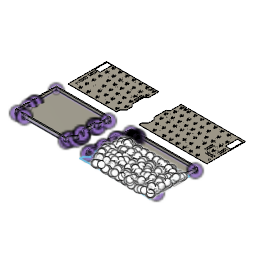
Keyboard Chassis Final v5 (Autodesk Fusion 360 design; units mm, degrees)
Autodesk Fusion 360 part; units mm, degrees
(part 1 of 12)
sketch "PCB_LEFT_MAIN" plane through (0, 0, 0) normal (0, 0, 1) x (1, 0, 0)
  line L0 (232.4105, -25.1856) -> (231.3945, -25.1856)
  line L1 (216.6624, -80.6847) -> (216.6624, -65.9527)
  line L2 (0, -1.9445) -> (0.127, -7.2798)
  line L3 (0, -79.6292) -> (0, -81.0262)
  line L4 (0, -81.0262) -> (30.2261, -80.6847)
  line L5 (231.3945, -25.1856) -> (222.2504, -16.0416)
  line L6 (0.127, -7.2798) -> (0, -32.8931)
  line L7 (222.2504, -16.0416) -> (222.2504, 39.8386)
  line L8 (233.4265, 46.9506) -> (233.4265, 92.0357)
  line L9 (226.3145, 39.8386) -> (233.4265, 46.9506)
  line L10 (222.2504, 39.8386) -> (226.3145, 39.8386)
  line L11 (232.4105, -50.2046) -> (232.4105, -25.1856)
  line L12 (233.4265, 92.0357) -> (0.635, 92.0357)
  line L13 (0.635, 92.0357) -> (0, 92.0357)
  line L14 (0, -69.7231) -> (0, -79.6292)
  line L15 (0, 92.0357) -> (0, -1.9445)
  line L16 (30.2261, -80.6847) -> (216.6624, -80.6847)
  line L17 (0, -32.8931) -> (0, -69.7231)
  line L18 (216.6624, -65.9527) -> (232.4105, -50.2046)
  line L19 (13.8092, -53.934) -> (12.9091, -53.934)
  line L20 (13.8092, -62.234) -> (12.9092, -62.234)
  line L21 (13.8092, -55.0339) -> (13.8092, -53.934)
  line L22 (13.8092, -61.1339) -> (13.8092, -62.234)
  line L23 (13.099, -61.1339) -> (13.8092, -61.1339)
  line L24 (13.8092, -55.0339) -> (13.1837, -55.0339)
  line L25 (13.1837, -55.0339) -> (13.1652, -55.0339)
  arc A0 (13.1652, -55.0339) -> (12.9092, -55.2899) centre (13.1653, -55.29) ccw
  line L26 (12.9092, -55.3429) -> (12.9092, -60.9441)
  arc A1 (12.9092, -60.9441) -> (13.099, -61.1339) centre (13.0991, -60.944) ccw
  arc A2 (13.8092, -54.1469) -> (13.8071, -54.149) centre (13.8071, -54.1469) cw
  line L27 (13.8092, -53.934) -> (12.9091, -53.934)
  line L28 (13.8092, -62.234) -> (12.9092, -62.234)
  line L29 (13.8092, -55.0339) -> (13.8092, -53.934)
  line L30 (13.8092, -61.1339) -> (13.8092, -62.234)
  line L31 (13.099, -61.1339) -> (13.8092, -61.1339)
  line L32 (13.8092, -55.0339) -> (13.1837, -55.0339)
  line L33 (13.1837, -55.0339) -> (13.1652, -55.0339)
  arc A3 (13.1652, -55.0339) -> (12.9092, -55.2899) centre (13.1653, -55.29) ccw
  line L34 (12.9092, -55.3429) -> (12.9092, -60.9441)
  arc A4 (12.9092, -60.9441) -> (13.099, -61.1339) centre (13.0991, -60.944) ccw
  arc A5 (13.8092, -54.1469) -> (13.8071, -54.149) centre (13.8071, -54.1469) cw
  arc A6 (39.6622, 82.1982) -> (43.65, 82.1982) centre (41.6561, 82.1982) ccw
  arc A7 (43.65, 82.1982) -> (39.6622, 82.1982) centre (41.6561, 82.1982) ccw
  arc A8 (47.587, 82.0712) -> (45.8852, 82.0712) centre (46.7361, 82.0712) ccw
  arc A9 (45.8852, 82.0712) -> (47.587, 82.0712) centre (46.7361, 82.0712) ccw
  arc A10 (37.427, 82.0712) -> (35.7252, 82.0712) centre (36.5761, 82.0712) ccw
  arc A11 (35.7252, 82.0712) -> (37.427, 82.0712) centre (36.5761, 82.0712) ccw
  arc A12 (69.6622, 82.1982) -> (73.65, 82.1982) centre (71.6561, 82.1982) ccw
  arc A13 (73.65, 82.1982) -> (69.6622, 82.1982) centre (71.6561, 82.1982) ccw
  arc A14 (77.587, 82.0712) -> (75.8852, 82.0712) centre (76.7361, 82.0712) ccw
  arc A15 (75.8852, 82.0712) -> (77.587, 82.0712) centre (76.7361, 82.0712) ccw
  arc A16 (65.7252, 82.0712) -> (67.427, 82.0712) centre (66.5761, 82.0712) ccw
  arc A17 (67.427, 82.0712) -> (65.7252, 82.0712) centre (66.5761, 82.0712) ccw
  arc A18 (99.6622, 82.1982) -> (103.65, 82.1982) centre (101.6561, 82.1982) ccw
  arc A19 (103.65, 82.1982) -> (99.6622, 82.1982) centre (101.6561, 82.1982) ccw
  arc A20 (107.587, 82.0712) -> (105.8852, 82.0712) centre (106.7361, 82.0712) ccw
  arc A21 (105.8852, 82.0712) -> (107.587, 82.0712) centre (106.7361, 82.0712) ccw
  arc A22 (95.7252, 82.0712) -> (97.427, 82.0712) centre (96.5761, 82.0712) ccw
  arc A23 (97.427, 82.0712) -> (95.7252, 82.0712) centre (96.5761, 82.0712) ccw
  arc A24 (133.65, 82.1982) -> (129.6622, 82.1982) centre (131.6561, 82.1982) ccw
  arc A25 (129.6622, 82.1982) -> (133.65, 82.1982) centre (131.6561, 82.1982) ccw
  arc A26 (135.8852, 82.0712) -> (137.587, 82.0712) centre (136.7361, 82.0712) ccw
  arc A27 (137.587, 82.0712) -> (135.8852, 82.0712) centre (136.7361, 82.0712) ccw
  arc A28 (125.7252, 82.0712) -> (127.427, 82.0712) centre (126.5761, 82.0712) ccw
  arc A29 (127.427, 82.0712) -> (125.7252, 82.0712) centre (126.5761, 82.0712) ccw
  arc A30 (163.65, 82.1982) -> (159.6622, 82.1982) centre (161.6561, 82.1982) ccw
  arc A31 (159.6622, 82.1982) -> (163.65, 82.1982) centre (161.6561, 82.1982) ccw
  arc A32 (167.587, 82.0712) -> (165.8852, 82.0712) centre (166.7361, 82.0712) ccw
  arc A33 (165.8852, 82.0712) -> (167.587, 82.0712) centre (166.7361, 82.0712) ccw
  arc A34 (155.7252, 82.0712) -> (157.427, 82.0712) centre (156.5761, 82.0712) ccw
  arc A35 (157.427, 82.0712) -> (155.7252, 82.0712) centre (156.5761, 82.0712) ccw
  arc A36 (193.65, 82.1982) -> (189.6622, 82.1982) centre (191.6561, 82.1982) ccw
  arc A37 (189.6622, 82.1982) -> (193.65, 82.1982) centre (191.6561, 82.1982) ccw
  arc A38 (197.587, 82.0712) -> (195.8852, 82.0712) centre (196.7361, 82.0712) ccw
  arc A39 (195.8852, 82.0712) -> (197.587, 82.0712) centre (196.7361, 82.0712) ccw
  arc A40 (187.427, 82.0712) -> (185.7252, 82.0712) centre (186.5761, 82.0712) ccw
  arc A41 (185.7252, 82.0712) -> (187.427, 82.0712) centre (186.5761, 82.0712) ccw
  arc A42 (223.65, 82.1982) -> (219.6622, 82.1982) centre (221.6561, 82.1982) ccw
  arc A43 (219.6622, 82.1982) -> (223.65, 82.1982) centre (221.6561, 82.1982) ccw
  arc A44 (227.587, 82.0712) -> (225.8852, 82.0712) centre (226.7361, 82.0712) ccw
  arc A45 (225.8852, 82.0712) -> (227.587, 82.0712) centre (226.7361, 82.0712) ccw
  arc A46 (215.7252, 82.0712) -> (217.427, 82.0712) centre (216.5761, 82.0712) ccw
  arc A47 (217.427, 82.0712) -> (215.7252, 82.0712) centre (216.5761, 82.0712) ccw
  arc A48 (39.6622, 52.1982) -> (43.65, 52.1982) centre (41.6561, 52.1982) ccw
  arc A49 (43.65, 52.1982) -> (39.6622, 52.1982) centre (41.6561, 52.1982) ccw
  arc A50 (47.587, 52.0712) -> (45.8852, 52.0712) centre (46.7361, 52.0712) ccw
  arc A51 (45.8852, 52.0712) -> (47.587, 52.0712) centre (46.7361, 52.0712) ccw
  arc A52 (37.427, 52.0712) -> (35.7252, 52.0712) centre (36.5761, 52.0712) ccw
  arc A53 (35.7252, 52.0712) -> (37.427, 52.0712) centre (36.5761, 52.0712) ccw
  arc A54 (73.65, 52.1982) -> (69.6622, 52.1982) centre (71.6561, 52.1982) ccw
  arc A55 (69.6622, 52.1982) -> (73.65, 52.1982) centre (71.6561, 52.1982) ccw
  arc A56 (75.8852, 52.0712) -> (77.587, 52.0712) centre (76.7361, 52.0712) ccw
  arc A57 (77.587, 52.0712) -> (75.8852, 52.0712) centre (76.7361, 52.0712) ccw
  arc A58 (67.427, 52.0712) -> (65.7252, 52.0712) centre (66.5761, 52.0712) ccw
  arc A59 (65.7252, 52.0712) -> (67.427, 52.0712) centre (66.5761, 52.0712) ccw
  arc A60 (103.65, 52.1982) -> (99.6622, 52.1982) centre (101.6561, 52.1982) ccw
  arc A61 (99.6622, 52.1982) -> (103.65, 52.1982) centre (101.6561, 52.1982) ccw
  arc A62 (105.8852, 52.0712) -> (107.587, 52.0712) centre (106.7361, 52.0712) ccw
  arc A63 (107.587, 52.0712) -> (105.8852, 52.0712) centre (106.7361, 52.0712) ccw
  arc A64 (97.427, 52.0712) -> (95.7252, 52.0712) centre (96.5761, 52.0712) ccw
  arc A65 (95.7252, 52.0712) -> (97.427, 52.0712) centre (96.5761, 52.0712) ccw
  arc A66 (133.65, 52.1982) -> (129.6622, 52.1982) centre (131.6561, 52.1982) ccw
  arc A67 (129.6622, 52.1982) -> (133.65, 52.1982) centre (131.6561, 52.1982) ccw
  arc A68 (137.587, 52.0712) -> (135.8852, 52.0712) centre (136.7361, 52.0712) ccw
  arc A69 (135.8852, 52.0712) -> (137.587, 52.0712) centre (136.7361, 52.0712) ccw
  arc A70 (127.427, 52.0712) -> (125.7252, 52.0712) centre (126.5761, 52.0712) ccw
  arc A71 (125.7252, 52.0712) -> (127.427, 52.0712) centre (126.5761, 52.0712) ccw
  arc A72 (159.6622, 52.1982) -> (163.65, 52.1982) centre (161.6561, 52.1982) ccw
  arc A73 (163.65, 52.1982) -> (159.6622, 52.1982) centre (161.6561, 52.1982) ccw
  arc A74 (165.8852, 52.0712) -> (167.587, 52.0712) centre (166.7361, 52.0712) ccw
  arc A75 (167.587, 52.0712) -> (165.8852, 52.0712) centre (166.7361, 52.0712) ccw
  arc A76 (155.7252, 52.0712) -> (157.427, 52.0712) centre (156.5761, 52.0712) ccw
  arc A77 (157.427, 52.0712) -> (155.7252, 52.0712) centre (156.5761, 52.0712) ccw
  arc A78 (193.65, 52.1982) -> (189.6622, 52.1982) centre (191.6561, 52.1982) ccw
  arc A79 (189.6622, 52.1982) -> (193.65, 52.1982) centre (191.6561, 52.1982) ccw
  arc A80 (197.587, 52.0712) -> (195.8852, 52.0712) centre (196.7361, 52.0712) ccw
  arc A81 (195.8852, 52.0712) -> (197.587, 52.0712) centre (196.7361, 52.0712) ccw
  arc A82 (185.7252, 52.0712) -> (187.427, 52.0712) centre (186.5761, 52.0712) ccw
  arc A83 (187.427, 52.0712) -> (185.7252, 52.0712) centre (186.5761, 52.0712) ccw
  arc A84 (219.6622, 52.1982) -> (223.65, 52.1982) centre (221.6561, 52.1982) ccw
  arc A85 (223.65, 52.1982) -> (219.6622, 52.1982) centre (221.6561, 52.1982) ccw
  arc A86 (225.8852, 52.0712) -> (227.587, 52.0712) centre (226.7361, 52.0712) ccw
  arc A87 (227.587, 52.0712) -> (225.8852, 52.0712) centre (226.7361, 52.0712) ccw
  arc A88 (217.427, 52.0712) -> (215.7252, 52.0712) centre (216.5761, 52.0712) ccw
  arc A89 (215.7252, 52.0712) -> (217.427, 52.0712) centre (216.5761, 52.0712) ccw
  arc A90 (43.65, 22.1982) -> (39.6622, 22.1982) centre (41.6561, 22.1982) ccw
  arc A91 (39.6622, 22.1982) -> (43.65, 22.1982) centre (41.6561, 22.1982) ccw
  arc A92 (45.8852, 22.0712) -> (47.587, 22.0712) centre (46.7361, 22.0712) ccw
  arc A93 (47.587, 22.0712) -> (45.8852, 22.0712) centre (46.7361, 22.0712) ccw
  arc A94 (37.427, 22.0712) -> (35.7252, 22.0712) centre (36.5761, 22.0712) ccw
  arc A95 (35.7252, 22.0712) -> (37.427, 22.0712) centre (36.5761, 22.0712) ccw
  arc A96 (75.7455, 22.2541) -> (79.7333, 22.2541) centre (77.7394, 22.2541) ccw
  arc A97 (79.7333, 22.2541) -> (75.7455, 22.2541) centre (77.7394, 22.2541) ccw
  arc A98 (83.6703, 22.1271) -> (81.9685, 22.1271) centre (82.8194, 22.1271) ccw
  arc A99 (81.9685, 22.1271) -> (83.6703, 22.1271) centre (82.8194, 22.1271) ccw
  arc A100 (73.5103, 22.1271) -> (71.8085, 22.1271) centre (72.6594, 22.1271) ccw
  arc A101 (71.8085, 22.1271) -> (73.5103, 22.1271) centre (72.6594, 22.1271) ccw
  arc A102 (105.7455, 22.2541) -> (109.7333, 22.2541) centre (107.7394, 22.2541) ccw
  arc A103 (109.7333, 22.2541) -> (105.7455, 22.2541) centre (107.7394, 22.2541) ccw
  arc A104 (111.9685, 22.1271) -> (113.6703, 22.1271) centre (112.8194, 22.1271) ccw
  arc A105 (113.6703, 22.1271) -> (111.9685, 22.1271) centre (112.8194, 22.1271) ccw
  arc A106 (101.8085, 22.1271) -> (103.5103, 22.1271) centre (102.6594, 22.1271) ccw
  arc A107 (103.5103, 22.1271) -> (101.8085, 22.1271) centre (102.6594, 22.1271) ccw
  arc A108 (135.7455, 22.2541) -> (139.7333, 22.2541) centre (137.7394, 22.2541) ccw
  arc A109 (139.7333, 22.2541) -> (135.7455, 22.2541) centre (137.7394, 22.2541) ccw
  arc A110 (143.6703, 22.1271) -> (141.9685, 22.1271) centre (142.8194, 22.1271) ccw
  arc A111 (141.9685, 22.1271) -> (143.6703, 22.1271) centre (142.8194, 22.1271) ccw
  arc A112 (133.5103, 22.1271) -> (131.8085, 22.1271) centre (132.6594, 22.1271) ccw
  arc A113 (131.8085, 22.1271) -> (133.5103, 22.1271) centre (132.6594, 22.1271) ccw
  arc A114 (165.7455, 22.2541) -> (169.7333, 22.2541) centre (167.7394, 22.2541) ccw
  arc A115 (169.7333, 22.2541) -> (165.7455, 22.2541) centre (167.7394, 22.2541) ccw
  arc A116 (173.6703, 22.1271) -> (171.9685, 22.1271) centre (172.8194, 22.1271) ccw
  arc A117 (171.9685, 22.1271) -> (173.6703, 22.1271) centre (172.8194, 22.1271) ccw
  arc A118 (163.5103, 22.1271) -> (161.8085, 22.1271) centre (162.6594, 22.1271) ccw
  arc A119 (161.8085, 22.1271) -> (163.5103, 22.1271) centre (162.6594, 22.1271) ccw
  arc A120 (199.7333, 22.2541) -> (195.7455, 22.2541) centre (197.7394, 22.2541) ccw
  arc A121 (195.7455, 22.2541) -> (199.7333, 22.2541) centre (197.7394, 22.2541) ccw
  arc A122 (203.6703, 22.1271) -> (201.9685, 22.1271) centre (202.8194, 22.1271) ccw
  arc A123 (201.9685, 22.1271) -> (203.6703, 22.1271) centre (202.8194, 22.1271) ccw
  arc A124 (193.5103, 22.1271) -> (191.8085, 22.1271) centre (192.6594, 22.1271) ccw
  arc A125 (191.8085, 22.1271) -> (193.5103, 22.1271) centre (192.6594, 22.1271) ccw
  arc A126 (118.4531, -65.1919) -> (114.4653, -65.1919) centre (116.4592, -65.1919) ccw
  arc A127 (114.4653, -65.1919) -> (118.4531, -65.1919) centre (116.4592, -65.1919) ccw
  arc A128 (122.3901, -65.3189) -> (120.6883, -65.3189) centre (121.5392, -65.3189) ccw
  arc A129 (120.6883, -65.3189) -> (122.3901, -65.3189) centre (121.5392, -65.3189) ccw
  arc A130 (112.2301, -65.3189) -> (110.5283, -65.3189) centre (111.3792, -65.3189) ccw
  arc A131 (110.5283, -65.3189) -> (112.2301, -65.3189) centre (111.3792, -65.3189) ccw
  arc A132 (39.6622, -7.8018) -> (43.65, -7.8018) centre (41.6561, -7.8018) ccw
  arc A133 (43.65, -7.8018) -> (39.6622, -7.8018) centre (41.6561, -7.8018) ccw
  arc A134 (47.587, -7.9288) -> (45.8852, -7.9288) centre (46.7361, -7.9288) ccw
  arc A135 (45.8852, -7.9288) -> (47.587, -7.9288) centre (46.7361, -7.9288) ccw
  arc A136 (37.427, -7.9288) -> (35.7252, -7.9288) centre (36.5761, -7.9288) ccw
  arc A137 (35.7252, -7.9288) -> (37.427, -7.9288) centre (36.5761, -7.9288) ccw
  arc A138 (86.6675, -7.845) -> (90.6553, -7.845) centre (88.6614, -7.845) ccw
  arc A139 (90.6553, -7.845) -> (86.6675, -7.845) centre (88.6614, -7.845) ccw
  arc A140 (94.5923, -7.972) -> (92.8905, -7.972) centre (93.7414, -7.972) ccw
  arc A141 (92.8905, -7.972) -> (94.5923, -7.972) centre (93.7414, -7.972) ccw
  arc A142 (84.4323, -7.972) -> (82.7305, -7.972) centre (83.5814, -7.972) ccw
  arc A143 (82.7305, -7.972) -> (84.4323, -7.972) centre (83.5814, -7.972) ccw
  arc A144 (116.6675, -7.845) -> (120.6553, -7.845) centre (118.6614, -7.845) ccw
  arc A145 (120.6553, -7.845) -> (116.6675, -7.845) centre (118.6614, -7.845) ccw
  arc A146 (122.8905, -7.972) -> (124.5923, -7.972) centre (123.7414, -7.972) ccw
  arc A147 (124.5923, -7.972) -> (122.8905, -7.972) centre (123.7414, -7.972) ccw
  arc A148 (112.7305, -7.972) -> (114.4323, -7.972) centre (113.5814, -7.972) ccw
  arc A149 (114.4323, -7.972) -> (112.7305, -7.972) centre (113.5814, -7.972) ccw
  arc A150 (146.6675, -7.845) -> (150.6553, -7.845) centre (148.6614, -7.845) ccw
  arc A151 (150.6553, -7.845) -> (146.6675, -7.845) centre (148.6614, -7.845) ccw
  arc A152 (154.5923, -7.972) -> (152.8905, -7.972) centre (153.7414, -7.972) ccw
  arc A153 (152.8905, -7.972) -> (154.5923, -7.972) centre (153.7414, -7.972) ccw
  arc A154 (142.7305, -7.972) -> (144.4323, -7.972) centre (143.5814, -7.972) ccw
  arc A155 (144.4323, -7.972) -> (142.7305, -7.972) centre (143.5814, -7.972) ccw
  arc A156 (176.6675, -7.845) -> (180.6553, -7.845) centre (178.6614, -7.845) ccw
  arc A157 (180.6553, -7.845) -> (176.6675, -7.845) centre (178.6614, -7.845) ccw
  arc A158 (184.5923, -7.972) -> (182.8905, -7.972) centre (183.7414, -7.972) ccw
  arc A159 (182.8905, -7.972) -> (184.5923, -7.972) centre (183.7414, -7.972) ccw
  arc A160 (174.4323, -7.972) -> (172.7305, -7.972) centre (173.5814, -7.972) ccw
  arc A161 (172.7305, -7.972) -> (174.4323, -7.972) centre (173.5814, -7.972) ccw
  arc A162 (210.6553, -7.845) -> (206.6675, -7.845) centre (208.6614, -7.845) ccw
  arc A163 (206.6675, -7.845) -> (210.6553, -7.845) centre (208.6614, -7.845) ccw
  arc A164 (212.8905, -7.972) -> (214.5923, -7.972) centre (213.7414, -7.972) ccw
  arc A165 (214.5923, -7.972) -> (212.8905, -7.972) centre (213.7414, -7.972) ccw
  arc A166 (202.7305, -7.972) -> (204.4323, -7.972) centre (203.5814, -7.972) ccw
  arc A167 (204.4323, -7.972) -> (202.7305, -7.972) centre (203.5814, -7.972) ccw
  arc A168 (158.5344, -65.1919) -> (162.5222, -65.1919) centre (160.5283, -65.1919) ccw
  arc A169 (162.5222, -65.1919) -> (158.5344, -65.1919) centre (160.5283, -65.1919) ccw
  arc A170 (166.4592, -65.3189) -> (164.7574, -65.3189) centre (165.6083, -65.3189) ccw
  arc A171 (164.7574, -65.3189) -> (166.4592, -65.3189) centre (165.6083, -65.3189) ccw
  arc A172 (156.2992, -65.3189) -> (154.5974, -65.3189) centre (155.4483, -65.3189) ccw
  arc A173 (154.5974, -65.3189) -> (156.2992, -65.3189) centre (155.4483, -65.3189) ccw
  arc A174 (39.6622, -37.8018) -> (43.65, -37.8018) centre (41.6561, -37.8018) ccw
  arc A175 (43.65, -37.8018) -> (39.6622, -37.8018) centre (41.6561, -37.8018) ccw
  arc A176 (47.587, -37.9288) -> (45.8852, -37.9288) centre (46.7361, -37.9288) ccw
  arc A177 (45.8852, -37.9288) -> (47.587, -37.9288) centre (46.7361, -37.9288) ccw
  arc A178 (37.427, -37.9288) -> (35.7252, -37.9288) centre (36.5761, -37.9288) ccw
  arc A179 (35.7252, -37.9288) -> (37.427, -37.9288) centre (36.5761, -37.9288) ccw
  arc A180 (100.1803, -37.817) -> (96.1925, -37.817) centre (98.1864, -37.817) ccw
  arc A181 (96.1925, -37.817) -> (100.1803, -37.817) centre (98.1864, -37.817) ccw
  arc A182 (102.4155, -37.944) -> (104.1173, -37.944) centre (103.2664, -37.944) ccw
  arc A183 (104.1173, -37.944) -> (102.4155, -37.944) centre (103.2664, -37.944) ccw
  arc A184 (92.2555, -37.944) -> (93.9573, -37.944) centre (93.1064, -37.944) ccw
  arc A185 (93.9573, -37.944) -> (92.2555, -37.944) centre (93.1064, -37.944) ccw
  arc A186 (130.1803, -37.817) -> (126.1925, -37.817) centre (128.1864, -37.817) ccw
  arc A187 (126.1925, -37.817) -> (130.1803, -37.817) centre (128.1864, -37.817) ccw
  arc A188 (132.4155, -37.944) -> (134.1173, -37.944) centre (133.2664, -37.944) ccw
  arc A189 (134.1173, -37.944) -> (132.4155, -37.944) centre (133.2664, -37.944) ccw
  arc A190 (122.2555, -37.944) -> (123.9573, -37.944) centre (123.1064, -37.944) ccw
  arc A191 (123.9573, -37.944) -> (122.2555, -37.944) centre (123.1064, -37.944) ccw
  arc A192 (156.1925, -37.817) -> (160.1803, -37.817) centre (158.1864, -37.817) ccw
  arc A193 (160.1803, -37.817) -> (156.1925, -37.817) centre (158.1864, -37.817) ccw
  arc A194 (162.4155, -37.944) -> (164.1173, -37.944) centre (163.2664, -37.944) ccw
  arc A195 (164.1173, -37.944) -> (162.4155, -37.944) centre (163.2664, -37.944) ccw
  arc A196 (153.9573, -37.944) -> (152.2555, -37.944) centre (153.1064, -37.944) ccw
  arc A197 (152.2555, -37.944) -> (153.9573, -37.944) centre (153.1064, -37.944) ccw
  arc A198 (190.1803, -37.817) -> (186.1925, -37.817) centre (188.1864, -37.817) ccw
  arc A199 (186.1925, -37.817) -> (190.1803, -37.817) centre (188.1864, -37.817) ccw
  arc A200 (192.4155, -37.944) -> (194.1173, -37.944) centre (193.2664, -37.944) ccw
  arc A201 (194.1173, -37.944) -> (192.4155, -37.944) centre (193.2664, -37.944) ccw
  arc A202 (183.9573, -37.944) -> (182.2555, -37.944) centre (183.1064, -37.944) ccw
  arc A203 (182.2555, -37.944) -> (183.9573, -37.944) centre (183.1064, -37.944) ccw
  arc A204 (220.1803, -37.817) -> (216.1925, -37.817) centre (218.1864, -37.817) ccw
  arc A205 (216.1925, -37.817) -> (220.1803, -37.817) centre (218.1864, -37.817) ccw
  arc A206 (222.4155, -37.944) -> (224.1173, -37.944) centre (223.2664, -37.944) ccw
  arc A207 (224.1173, -37.944) -> (222.4155, -37.944) centre (223.2664, -37.944) ccw
  arc A208 (213.9573, -37.944) -> (212.2555, -37.944) centre (213.1064, -37.944) ccw
  arc A209 (212.2555, -37.944) -> (213.9573, -37.944) centre (213.1064, -37.944) ccw
  arc A210 (206.9723, -65.1919) -> (202.9845, -65.1919) centre (204.9784, -65.1919) ccw
  arc A211 (202.9845, -65.1919) -> (206.9723, -65.1919) centre (204.9784, -65.1919) ccw
  arc A212 (209.2075, -65.3189) -> (210.9093, -65.3189) centre (210.0584, -65.3189) ccw
  arc A213 (210.9093, -65.3189) -> (209.2075, -65.3189) centre (210.0584, -65.3189) ccw
  arc A214 (200.7493, -65.3189) -> (199.0475, -65.3189) centre (199.8984, -65.3189) ccw
  arc A215 (199.0475, -65.3189) -> (200.7493, -65.3189) centre (199.8984, -65.3189) ccw
  arc A216 (39.6622, -65.1919) -> (43.65, -65.1919) centre (41.6561, -65.1919) ccw
  arc A217 (43.65, -65.1919) -> (39.6622, -65.1919) centre (41.6561, -65.1919) ccw
  arc A218 (45.8852, -65.3189) -> (47.587, -65.3189) centre (46.7361, -65.3189) ccw
  arc A219 (47.587, -65.3189) -> (45.8852, -65.3189) centre (46.7361, -65.3189) ccw
  arc A220 (35.7252, -65.3189) -> (37.427, -65.3189) centre (36.5761, -65.3189) ccw
  arc A221 (37.427, -65.3189) -> (35.7252, -65.3189) centre (36.5761, -65.3189) ccw
  arc A222 (73.8252, -65.1919) -> (77.8131, -65.1919) centre (75.8192, -65.1919) ccw
  arc A223 (77.8131, -65.1919) -> (73.8252, -65.1919) centre (75.8192, -65.1919) ccw
  arc A224 (80.0483, -65.3189) -> (81.7501, -65.3189) centre (80.8992, -65.3189) ccw
  arc A225 (81.7501, -65.3189) -> (80.0483, -65.3189) centre (80.8992, -65.3189) ccw
  arc A226 (71.59, -65.3189) -> (69.8882, -65.3189) centre (70.7391, -65.3189) ccw
  arc A227 (69.8882, -65.3189) -> (71.59, -65.3189) centre (70.7391, -65.3189) ccw
  arc A228 (207.6588, 87.4842) -> (206.1588, 87.4842) centre (206.9088, 87.4842) ccw
  arc A229 (206.1588, 87.4842) -> (207.6588, 87.4842) centre (206.9088, 87.4842) ccw
  arc A230 (207.7096, 80.4662) -> (206.2096, 80.4662) centre (206.9596, 80.4662) ccw
  arc A231 (206.2096, 80.4662) -> (207.7096, 80.4662) centre (206.9596, 80.4662) ccw
  line L35 (43.6781, 75.6042) -> (39.8781, 75.6042)
  line L36 (39.8781, 79.4042) -> (43.6781, 79.4042)
  line L37 (43.6781, 79.4042) -> (43.6781, 75.6042)
  line L38 (39.8781, 75.6042) -> (39.8781, 79.4042)
  line L39 (69.8781, 79.4042) -> (73.6781, 79.4042)
  line L40 (69.8781, 75.6042) -> (69.8781, 79.4042)
  line L41 (73.6781, 75.6042) -> (69.8781, 75.6042)
  line L42 (73.6781, 79.4042) -> (73.6781, 75.6042)
  line L43 (99.8781, 79.4042) -> (103.6781, 79.4042)
  line L44 (103.6781, 75.6042) -> (99.8781, 75.6042)
  line L45 (103.6781, 79.4042) -> (103.6781, 75.6042)
  line L46 (99.8781, 75.6042) -> (99.8781, 79.4042)
  line L47 (129.8781, 79.4042) -> (133.6781, 79.4042)
  line L48 (129.8781, 75.6042) -> (129.8781, 79.4042)
  line L49 (133.6781, 79.4042) -> (133.6781, 75.6042)
  line L50 (133.6781, 75.6042) -> (129.8781, 75.6042)
  line L51 (163.6781, 75.6042) -> (159.8781, 75.6042)
  line L52 (159.8781, 79.4042) -> (163.6781, 79.4042)
  line L53 (159.8781, 75.6042) -> (159.8781, 79.4042)
  line L54 (163.6781, 79.4042) -> (163.6781, 75.6042)
  line L55 (189.8781, 75.6042) -> (189.8781, 79.4042)
  line L56 (193.6781, 75.6042) -> (189.8781, 75.6042)
  line L57 (193.6781, 79.4042) -> (193.6781, 75.6042)
  line L58 (189.8781, 79.4042) -> (193.6781, 79.4042)
  line L59 (219.8781, 75.6042) -> (219.8781, 79.4042)
  line L60 (223.6781, 75.6042) -> (219.8781, 75.6042)
  line L61 (223.6781, 79.4042) -> (223.6781, 75.6042)
  line L62 (219.8781, 79.4042) -> (223.6781, 79.4042)
  line L63 (43.6781, 45.6042) -> (39.8781, 45.6042)
  line L64 (43.6781, 49.4042) -> (43.6781, 45.6042)
  line L65 (39.8781, 49.4042) -> (43.6781, 49.4042)
  line L66 (39.8781, 45.6042) -> (39.8781, 49.4042)
  line L67 (73.6781, 49.4042) -> (73.6781, 45.6042)
  line L68 (69.8781, 45.6042) -> (69.8781, 49.4042)
  line L69 (69.8781, 49.4042) -> (73.6781, 49.4042)
  line L70 (73.6781, 45.6042) -> (69.8781, 45.6042)
  line L71 (103.6781, 49.4042) -> (103.6781, 45.6042)
  line L72 (99.8781, 49.4042) -> (103.6781, 49.4042)
  line L73 (99.8781, 45.6042) -> (99.8781, 49.4042)
  line L74 (103.6781, 45.6042) -> (99.8781, 45.6042)
  line L75 (129.8781, 45.6042) -> (129.8781, 49.4042)
  line L76 (133.6781, 49.4042) -> (133.6781, 45.6042)
  line L77 (133.6781, 45.6042) -> (129.8781, 45.6042)
  line L78 (129.8781, 49.4042) -> (133.6781, 49.4042)
  line L79 (159.8781, 49.4042) -> (163.6781, 49.4042)
  line L80 (163.6781, 45.6042) -> (159.8781, 45.6042)
  line L81 (159.8781, 45.6042) -> (159.8781, 49.4042)
  line L82 (163.6781, 49.4042) -> (163.6781, 45.6042)
  line L83 (189.8781, 45.6042) -> (189.8781, 49.4042)
  line L84 (193.6781, 45.6042) -> (189.8781, 45.6042)
  line L85 (189.8781, 49.4042) -> (193.6781, 49.4042)
  line L86 (193.6781, 49.4042) -> (193.6781, 45.6042)
  line L87 (223.6781, 45.6042) -> (219.8781, 45.6042)
  line L88 (219.8781, 45.6042) -> (219.8781, 49.4042)
  line L89 (223.6781, 49.4042) -> (223.6781, 45.6042)
  line L90 (219.8781, 49.4042) -> (223.6781, 49.4042)
  line L91 (43.6781, 19.4042) -> (43.6781, 15.6042)
  line L92 (39.8781, 15.6042) -> (39.8781, 19.4042)
  line L93 (43.6781, 15.6042) -> (39.8781, 15.6042)
  line L94 (39.8781, 19.4042) -> (43.6781, 19.4042)
  line L95 (75.9614, 19.4601) -> (79.7614, 19.4601)
  line L96 (79.7614, 19.4601) -> (79.7614, 15.6601)
  line L97 (79.7614, 15.6601) -> (75.9614, 15.6601)
  line L98 (75.9614, 15.6601) -> (75.9614, 19.4601)
  line L99 (109.7614, 15.6601) -> (105.9614, 15.6601)
  line L100 (105.9614, 15.6601) -> (105.9614, 19.4601)
  line L101 (109.7614, 19.4601) -> (109.7614, 15.6601)
  line L102 (105.9614, 19.4601) -> (109.7614, 19.4601)
  line L103 (135.9614, 15.6601) -> (135.9614, 19.4601)
  line L104 (139.7614, 19.4601) -> (139.7614, 15.6601)
  line L105 (139.7614, 15.6601) -> (135.9614, 15.6601)
  line L106 (135.9614, 19.4601) -> (139.7614, 19.4601)
  line L107 (165.9614, 15.6601) -> (165.9614, 19.4601)
  line L108 (169.7614, 15.6601) -> (165.9614, 15.6601)
  line L109 (169.7614, 19.4601) -> (169.7614, 15.6601)
  line L110 (165.9614, 19.4601) -> (169.7614, 19.4601)
  line L111 (199.7614, 15.6601) -> (195.9614, 15.6601)
  line L112 (195.9614, 19.4601) -> (199.7614, 19.4601)
  line L113 (195.9614, 15.6601) -> (195.9614, 19.4601)
  line L114 (199.7614, 19.4601) -> (199.7614, 15.6601)
  line L115 (114.6812, -67.9859) -> (118.4812, -67.9859)
  line L116 (114.6812, -71.7859) -> (114.6812, -67.9859)
  line L117 (118.4812, -71.7859) -> (114.6812, -71.7859)
  line L118 (118.4812, -67.9859) -> (118.4812, -71.7859)
  line L119 (39.8781, -14.3958) -> (39.8781, -10.5958)
  line L120 (43.6781, -14.3958) -> (39.8781, -14.3958)
  line L121 (43.6781, -10.5958) -> (43.6781, -14.3958)
  line L122 (39.8781, -10.5958) -> (43.6781, -10.5958)
  line L123 (86.8834, -14.439) -> (86.8834, -10.639)
  line L124 (90.6834, -14.439) -> (86.8834, -14.439)
  line L125 (86.8834, -10.639) -> (90.6834, -10.639)
  line L126 (90.6834, -10.639) -> (90.6834, -14.439)
  line L127 (120.6834, -10.639) -> (120.6834, -14.439)
  line L128 (116.8834, -14.439) -> (116.8834, -10.639)
  line L129 (120.6834, -14.439) -> (116.8834, -14.439)
  line L130 (116.8834, -10.639) -> (120.6834, -10.639)
  line L131 (146.8834, -14.439) -> (146.8834, -10.639)
  line L132 (150.6834, -10.639) -> (150.6834, -14.439)
  line L133 (146.8834, -10.639) -> (150.6834, -10.639)
  line L134 (150.6834, -14.439) -> (146.8834, -14.439)
  line L135 (180.6834, -14.439) -> (176.8834, -14.439)
  line L136 (180.6834, -10.639) -> (180.6834, -14.439)
  line L137 (176.8834, -10.639) -> (180.6834, -10.639)
  line L138 (176.8834, -14.439) -> (176.8834, -10.639)
  line L139 (206.8834, -14.439) -> (206.8834, -10.639)
  line L140 (206.8834, -10.639) -> (210.6834, -10.639)
  line L141 (210.6834, -10.639) -> (210.6834, -14.439)
  line L142 (210.6834, -14.439) -> (206.8834, -14.439)
  line L143 (158.7503, -67.9859) -> (162.5503, -67.9859)
  line L144 (158.7503, -71.7859) -> (158.7503, -67.9859)
  line L145 (162.5503, -71.7859) -> (158.7503, -71.7859)
  line L146 (162.5503, -67.9859) -> (162.5503, -71.7859)
  line L147 (39.8781, -44.3958) -> (39.8781, -40.5958)
  line L148 (43.6781, -40.5958) -> (43.6781, -44.3958)
  line L149 (43.6781, -44.3958) -> (39.8781, -44.3958)
  line L150 (39.8781, -40.5958) -> (43.6781, -40.5958)
  line L151 (96.4084, -44.411) -> (96.4084, -40.611)
  line L152 (100.2084, -40.611) -> (100.2084, -44.411)
  line L153 (100.2084, -44.411) -> (96.4084, -44.411)
  line L154 (96.4084, -40.611) -> (100.2084, -40.611)
  line L155 (126.4084, -44.411) -> (126.4084, -40.611)
  line L156 (130.2084, -44.411) -> (126.4084, -44.411)
  line L157 (126.4084, -40.611) -> (130.2084, -40.611)
  line L158 (130.2084, -40.611) -> (130.2084, -44.411)
  line L159 (156.4084, -40.611) -> (160.2084, -40.611)
  line L160 (160.2084, -44.411) -> (156.4084, -44.411)
  line L161 (156.4084, -44.411) -> (156.4084, -40.611)
  line L162 (160.2084, -40.611) -> (160.2084, -44.411)
  line L163 (190.2084, -44.411) -> (186.4084, -44.411)
  line L164 (186.4084, -44.411) -> (186.4084, -40.611)
  line L165 (186.4084, -40.611) -> (190.2084, -40.611)
  line L166 (190.2084, -40.611) -> (190.2084, -44.411)
  line L167 (216.4084, -44.411) -> (216.4084, -40.611)
  line L168 (220.2084, -44.411) -> (216.4084, -44.411)
  line L169 (220.2084, -40.611) -> (220.2084, -44.411)
  line L170 (216.4084, -40.611) -> (220.2084, -40.611)
  line L171 (207.0004, -67.9859) -> (207.0004, -71.7859)
  line L172 (203.2004, -67.9859) -> (207.0004, -67.9859)
  line L173 (207.0004, -71.7859) -> (203.2004, -71.7859)
  line L174 (203.2004, -71.7859) -> (203.2004, -67.9859)
  line L175 (39.8781, -67.9859) -> (43.6781, -67.9859)
  line L176 (43.6781, -67.9859) -> (43.6781, -71.7859)
  line L177 (43.6781, -71.7859) -> (39.8781, -71.7859)
  line L178 (39.8781, -71.7859) -> (39.8781, -67.9859)
  line L179 (77.8411, -67.9859) -> (77.8411, -71.7859)
  line L180 (74.0411, -71.7859) -> (74.0411, -67.9859)
  line L181 (77.8411, -71.7859) -> (74.0411, -71.7859)
  line L182 (74.0411, -67.9859) -> (77.8411, -67.9859)
  line L183 (7.15, 86.5354) -> (5.55, 86.5354)
  line L184 (7.15, 88.1354) -> (7.15, 86.5354)
  line L185 (5.55, 88.1354) -> (7.15, 88.1354)
  line L186 (5.55, 86.5354) -> (5.55, 88.1354)
  line L187 (5.55, 88.1354) -> (7.15, 88.1354)
  line L188 (5.55, 86.5354) -> (5.55, 88.1354)
  line L189 (7.15, 88.1354) -> (7.15, 86.5354)
  line L190 (7.15, 86.5354) -> (5.55, 86.5354)
  line L191 (5.55, 86.5354) -> (5.55, 88.1354)
  line L192 (5.55, 88.1354) -> (7.15, 88.1354)
  line L193 (7.15, 88.1354) -> (7.15, 86.5354)
  line L194 (7.15, 86.5354) -> (5.55, 86.5354)
  arc A232 (5.55, 84.7954) -> (7.15, 84.7954) centre (6.35, 84.7954) ccw
  arc A233 (7.15, 84.7954) -> (5.55, 84.7954) centre (6.35, 84.7954) ccw
  arc A234 (5.55, 84.7954) -> (7.15, 84.7954) centre (6.35, 84.7954) ccw
  arc A235 (7.15, 84.7954) -> (5.55, 84.7954) centre (6.35, 84.7954) ccw
  arc A236 (5.55, 84.7954) -> (7.15, 84.7954) centre (6.35, 84.7954) ccw
  arc A237 (7.15, 84.7954) -> (5.55, 84.7954) centre (6.35, 84.7954) ccw
  arc A238 (5.55, 82.2554) -> (7.15, 82.2554) centre (6.35, 82.2554) ccw
  arc A239 (7.15, 82.2554) -> (5.55, 82.2554) centre (6.35, 82.2554) ccw
  arc A240 (5.55, 82.2554) -> (7.15, 82.2554) centre (6.35, 82.2554) ccw
  arc A241 (7.15, 82.2554) -> (5.55, 82.2554) centre (6.35, 82.2554) ccw
  arc A242 (5.55, 82.2554) -> (7.15, 82.2554) centre (6.35, 82.2554) ccw
  arc A243 (7.15, 82.2554) -> (5.55, 82.2554) centre (6.35, 82.2554) ccw
  arc A244 (5.55, 79.7154) -> (7.15, 79.7154) centre (6.35, 79.7154) ccw
  arc A245 (7.15, 79.7154) -> (5.55, 79.7154) centre (6.35, 79.7154) ccw
  arc A246 (5.55, 79.7154) -> (7.15, 79.7154) centre (6.35, 79.7154) ccw
  arc A247 (7.15, 79.7154) -> (5.55, 79.7154) centre (6.35, 79.7154) ccw
  arc A248 (7.15, 79.7154) -> (5.55, 79.7154) centre (6.35, 79.7154) ccw
  arc A249 (5.55, 79.7154) -> (7.15, 79.7154) centre (6.35, 79.7154) ccw
  arc A250 (7.15, 77.1754) -> (5.55, 77.1754) centre (6.35, 77.1754) ccw
  arc A251 (5.55, 77.1754) -> (7.15, 77.1754) centre (6.35, 77.1754) ccw
  arc A252 (7.15, 77.1754) -> (5.55, 77.1754) centre (6.35, 77.1754) ccw
  arc A253 (5.55, 77.1754) -> (7.15, 77.1754) centre (6.35, 77.1754) ccw
  arc A254 (5.55, 77.1754) -> (7.15, 77.1754) centre (6.35, 77.1754) ccw
  arc A255 (7.15, 77.1754) -> (5.55, 77.1754) centre (6.35, 77.1754) ccw
  arc A256 (7.15, 74.6354) -> (5.55, 74.6354) centre (6.35, 74.6354) ccw
  arc A257 (5.55, 74.6354) -> (7.15, 74.6354) centre (6.35, 74.6354) ccw
  arc A258 (7.15, 74.6354) -> (5.55, 74.6354) centre (6.35, 74.6354) ccw
  arc A259 (5.55, 74.6354) -> (7.15, 74.6354) centre (6.35, 74.6354) ccw
  arc A260 (5.55, 74.6354) -> (7.15, 74.6354) centre (6.35, 74.6354) ccw
  arc A261 (7.15, 74.6354) -> (5.55, 74.6354) centre (6.35, 74.6354) ccw
  arc A262 (5.55, 72.0954) -> (7.15, 72.0954) centre (6.35, 72.0954) ccw
  arc A263 (7.15, 72.0954) -> (5.55, 72.0954) centre (6.35, 72.0954) ccw
  arc A264 (5.55, 72.0954) -> (7.15, 72.0954) centre (6.35, 72.0954) ccw
  arc A265 (7.15, 72.0954) -> (5.55, 72.0954) centre (6.35, 72.0954) ccw
  arc A266 (7.15, 72.0954) -> (5.55, 72.0954) centre (6.35, 72.0954) ccw
  arc A267 (5.55, 72.0954) -> (7.15, 72.0954) centre (6.35, 72.0954) ccw
  arc A268 (5.55, 69.5553) -> (7.15, 69.5553) centre (6.35, 69.5553) ccw
  arc A269 (7.15, 69.5553) -> (5.55, 69.5553) centre (6.35, 69.5553) ccw
  arc A270 (5.55, 69.5553) -> (7.15, 69.5553) centre (6.35, 69.5553) ccw
  arc A271 (7.15, 69.5553) -> (5.55, 69.5553) centre (6.35, 69.5553) ccw
  arc A272 (7.15, 69.5553) -> (5.55, 69.5553) centre (6.35, 69.5553) ccw
  arc A273 (5.55, 69.5553) -> (7.15, 69.5553) centre (6.35, 69.5553) ccw
  arc A274 (7.15, 67.0153) -> (5.55, 67.0153) centre (6.35, 67.0153) ccw
  arc A275 (5.55, 67.0153) -> (7.15, 67.0153) centre (6.35, 67.0153) ccw
  arc A276 (7.15, 67.0153) -> (5.55, 67.0153) centre (6.35, 67.0153) ccw
  arc A277 (5.55, 67.0153) -> (7.15, 67.0153) centre (6.35, 67.0153) ccw
  arc A278 (7.15, 67.0153) -> (5.55, 67.0153) centre (6.35, 67.0153) ccw
  arc A279 (5.55, 67.0153) -> (7.15, 67.0153) centre (6.35, 67.0153) ccw
  arc A280 (5.55, 64.4753) -> (7.15, 64.4753) centre (6.35, 64.4753) ccw
  arc A281 (7.15, 64.4753) -> (5.55, 64.4753) centre (6.35, 64.4753) ccw
  arc A282 (5.55, 64.4753) -> (7.15, 64.4753) centre (6.35, 64.4753) ccw
  arc A283 (7.15, 64.4753) -> (5.55, 64.4753) centre (6.35, 64.4753) ccw
  arc A284 (7.15, 64.4753) -> (5.55, 64.4753) centre (6.35, 64.4753) ccw
  arc A285 (5.55, 64.4753) -> (7.15, 64.4753) centre (6.35, 64.4753) ccw
  arc A286 (5.55, 61.9353) -> (7.15, 61.9353) centre (6.35, 61.9353) ccw
  arc A287 (7.15, 61.9353) -> (5.55, 61.9353) centre (6.35, 61.9353) ccw
  arc A288 (5.55, 61.9353) -> (7.15, 61.9353) centre (6.35, 61.9353) ccw
  arc A289 (7.15, 61.9353) -> (5.55, 61.9353) centre (6.35, 61.9353) ccw
  arc A290 (7.15, 61.9353) -> (5.55, 61.9353) centre (6.35, 61.9353) ccw
  arc A291 (5.55, 61.9353) -> (7.15, 61.9353) centre (6.35, 61.9353) ccw
  arc A292 (5.55, 59.3953) -> (7.15, 59.3953) centre (6.35, 59.3953) ccw
  arc A293 (7.15, 59.3953) -> (5.55, 59.3953) centre (6.35, 59.3953) ccw
  arc A294 (5.55, 59.3953) -> (7.15, 59.3953) centre (6.35, 59.3953) ccw
  arc A295 (7.15, 59.3953) -> (5.55, 59.3953) centre (6.35, 59.3953) ccw
  arc A296 (7.15, 59.3953) -> (5.55, 59.3953) centre (6.35, 59.3953) ccw
  arc A297 (5.55, 59.3953) -> (7.15, 59.3953) centre (6.35, 59.3953) ccw
  arc A298 (5.55, 56.8553) -> (7.15, 56.8553) centre (6.35, 56.8553) ccw
  arc A299 (7.15, 56.8553) -> (5.55, 56.8553) centre (6.35, 56.8553) ccw
  arc A300 (7.15, 56.8553) -> (5.55, 56.8553) centre (6.35, 56.8553) ccw
  arc A301 (5.55, 56.8553) -> (7.15, 56.8553) centre (6.35, 56.8553) ccw
  arc A302 (5.55, 56.8553) -> (7.15, 56.8553) centre (6.35, 56.8553) ccw
  arc A303 (7.15, 56.8553) -> (5.55, 56.8553) centre (6.35, 56.8553) ccw
  arc A304 (5.55, 54.3153) -> (7.15, 54.3153) centre (6.35, 54.3153) ccw
  arc A305 (7.15, 54.3153) -> (5.55, 54.3153) centre (6.35, 54.3153) ccw
  arc A306 (7.15, 54.3153) -> (5.55, 54.3153) centre (6.35, 54.3153) ccw
  arc A307 (5.55, 54.3153) -> (7.15, 54.3153) centre (6.35, 54.3153) ccw
  arc A308 (5.55, 54.3153) -> (7.15, 54.3153) centre (6.35, 54.3153) ccw
  arc A309 (7.15, 54.3153) -> (5.55, 54.3153) centre (6.35, 54.3153) ccw
  arc A310 (5.55, 51.7753) -> (7.15, 51.7753) centre (6.35, 51.7753) ccw
  arc A311 (7.15, 51.7753) -> (5.55, 51.7753) centre (6.35, 51.7753) ccw
  arc A312 (7.15, 51.7753) -> (5.55, 51.7753) centre (6.35, 51.7753) ccw
  arc A313 (5.55, 51.7753) -> (7.15, 51.7753) centre (6.35, 51.7753) ccw
  arc A314 (5.55, 51.7753) -> (7.15, 51.7753) centre (6.35, 51.7753) ccw
  arc A315 (7.15, 51.7753) -> (5.55, 51.7753) centre (6.35, 51.7753) ccw
  arc A316 (5.55, 49.2353) -> (7.15, 49.2353) centre (6.35, 49.2353) ccw
  arc A317 (7.15, 49.2353) -> (5.55, 49.2353) centre (6.35, 49.2353) ccw
  arc A318 (5.55, 49.2353) -> (7.15, 49.2353) centre (6.35, 49.2353) ccw
  arc A319 (7.15, 49.2353) -> (5.55, 49.2353) centre (6.35, 49.2353) ccw
  arc A320 (7.15, 49.2353) -> (5.55, 49.2353) centre (6.35, 49.2353) ccw
  arc A321 (5.55, 49.2353) -> (7.15, 49.2353) centre (6.35, 49.2353) ccw
  arc A322 (5.5426, 46.6991) -> (7.1426, 46.6991) centre (6.3426, 46.6991) ccw
  arc A323 (7.1426, 46.6991) -> (5.5426, 46.6991) centre (6.3426, 46.6991) ccw
  arc A324 (7.1426, 46.6991) -> (5.5426, 46.6991) centre (6.3426, 46.6991) ccw
  arc A325 (5.5426, 46.6991) -> (7.1426, 46.6991) centre (6.3426, 46.6991) ccw
  arc A326 (7.1426, 46.6991) -> (5.5426, 46.6991) centre (6.3426, 46.6991) ccw
  arc A327 (5.5426, 46.6991) -> (7.1426, 46.6991) centre (6.3426, 46.6991) ccw
  arc A328 (7.15, 44.1553) -> (5.55, 44.1553) centre (6.35, 44.1553) ccw
  arc A329 (5.55, 44.1553) -> (7.15, 44.1553) centre (6.35, 44.1553) ccw
  arc A330 (7.15, 44.1553) -> (5.55, 44.1553) centre (6.35, 44.1553) ccw
  arc A331 (5.55, 44.1553) -> (7.15, 44.1553) centre (6.35, 44.1553) ccw
  arc A332 (7.15, 44.1553) -> (5.55, 44.1553) centre (6.35, 44.1553) ccw
  arc A333 (5.55, 44.1553) -> (7.15, 44.1553) centre (6.35, 44.1553) ccw
  arc A334 (5.55, 41.6153) -> (7.15, 41.6153) centre (6.35, 41.6153) ccw
  arc A335 (7.15, 41.6153) -> (5.55, 41.6153) centre (6.35, 41.6153) ccw
  arc A336 (5.55, 41.6153) -> (7.15, 41.6153) centre (6.35, 41.6153) ccw
  arc A337 (7.15, 41.6153) -> (5.55, 41.6153) centre (6.35, 41.6153) ccw
  arc A338 (5.55, 41.6153) -> (7.15, 41.6153) centre (6.35, 41.6153) ccw
  arc A339 (7.15, 41.6153) -> (5.55, 41.6153) centre (6.35, 41.6153) ccw
  arc A340 (5.55, 39.0753) -> (7.15, 39.0753) centre (6.35, 39.0753) ccw
  arc A341 (7.15, 39.0753) -> (5.55, 39.0753) centre (6.35, 39.0753) ccw
  arc A342 (5.55, 39.0753) -> (7.15, 39.0753) centre (6.35, 39.0753) ccw
  arc A343 (7.15, 39.0753) -> (5.55, 39.0753) centre (6.35, 39.0753) ccw
  arc A344 (5.55, 39.0753) -> (7.15, 39.0753) centre (6.35, 39.0753) ccw
  arc A345 (7.15, 39.0753) -> (5.55, 39.0753) centre (6.35, 39.0753) ccw
  arc A346 (24.93, 39.0753) -> (23.33, 39.0753) centre (24.13, 39.0753) ccw
  arc A347 (23.33, 39.0753) -> (24.93, 39.0753) centre (24.13, 39.0753) ccw
  arc A348 (24.93, 39.0753) -> (23.33, 39.0753) centre (24.13, 39.0753) ccw
  arc A349 (23.33, 39.0753) -> (24.93, 39.0753) centre (24.13, 39.0753) ccw
  arc A350 (24.93, 39.0753) -> (23.33, 39.0753) centre (24.13, 39.0753) ccw
  arc A351 (23.33, 39.0753) -> (24.93, 39.0753) centre (24.13, 39.0753) ccw
  arc A352 (24.93, 41.6153) -> (23.33, 41.6153) centre (24.13, 41.6153) ccw
  arc A353 (23.33, 41.6153) -> (24.93, 41.6153) centre (24.13, 41.6153) ccw
  arc A354 (23.33, 41.6153) -> (24.93, 41.6153) centre (24.13, 41.6153) ccw
  arc A355 (24.93, 41.6153) -> (23.33, 41.6153) centre (24.13, 41.6153) ccw
  arc A356 (24.93, 41.6153) -> (23.33, 41.6153) centre (24.13, 41.6153) ccw
  arc A357 (23.33, 41.6153) -> (24.93, 41.6153) centre (24.13, 41.6153) ccw
  arc A358 (23.33, 44.0837) -> (24.93, 44.0837) centre (24.13, 44.0837) ccw
  arc A359 (24.93, 44.0837) -> (23.33, 44.0837) centre (24.13, 44.0837) ccw
  arc A360 (24.93, 44.0837) -> (23.33, 44.0837) centre (24.13, 44.0837) ccw
  arc A361 (23.33, 44.0837) -> (24.93, 44.0837) centre (24.13, 44.0837) ccw
  arc A362 (23.33, 44.0837) -> (24.93, 44.0837) centre (24.13, 44.0837) ccw
  arc A363 (24.93, 44.0837) -> (23.33, 44.0837) centre (24.13, 44.0837) ccw
  arc A364 (24.93, 46.6953) -> (23.33, 46.6953) centre (24.13, 46.6953) ccw
  arc A365 (23.33, 46.6953) -> (24.93, 46.6953) centre (24.13, 46.6953) ccw
  arc A366 (23.33, 46.6953) -> (24.93, 46.6953) centre (24.13, 46.6953) ccw
  arc A367 (24.93, 46.6953) -> (23.33, 46.6953) centre (24.13, 46.6953) ccw
  arc A368 (24.93, 46.6953) -> (23.33, 46.6953) centre (24.13, 46.6953) ccw
  arc A369 (23.33, 46.6953) -> (24.93, 46.6953) centre (24.13, 46.6953) ccw
  arc A370 (24.93, 49.2353) -> (23.33, 49.2353) centre (24.13, 49.2353) ccw
  arc A371 (23.33, 49.2353) -> (24.93, 49.2353) centre (24.13, 49.2353) ccw
  arc A372 (24.93, 49.2353) -> (23.33, 49.2353) centre (24.13, 49.2353) ccw
  arc A373 (23.33, 49.2353) -> (24.93, 49.2353) centre (24.13, 49.2353) ccw
  arc A374 (24.93, 49.2353) -> (23.33, 49.2353) centre (24.13, 49.2353) ccw
  arc A375 (23.33, 49.2353) -> (24.93, 49.2353) centre (24.13, 49.2353) ccw
  arc A376 (23.33, 51.7753) -> (24.93, 51.7753) centre (24.13, 51.7753) ccw
  arc A377 (24.93, 51.7753) -> (23.33, 51.7753) centre (24.13, 51.7753) ccw
  arc A378 (23.33, 51.7753) -> (24.93, 51.7753) centre (24.13, 51.7753) ccw
  arc A379 (24.93, 51.7753) -> (23.33, 51.7753) centre (24.13, 51.7753) ccw
  arc A380 (24.93, 51.7753) -> (23.33, 51.7753) centre (24.13, 51.7753) ccw
  arc A381 (23.33, 51.7753) -> (24.93, 51.7753) centre (24.13, 51.7753) ccw
  arc A382 (24.93, 54.3153) -> (23.33, 54.3153) centre (24.13, 54.3153) ccw
  arc A383 (23.33, 54.3153) -> (24.93, 54.3153) centre (24.13, 54.3153) ccw
  arc A384 (24.93, 54.3153) -> (23.33, 54.3153) centre (24.13, 54.3153) ccw
  arc A385 (23.33, 54.3153) -> (24.93, 54.3153) centre (24.13, 54.3153) ccw
  arc A386 (24.93, 54.3153) -> (23.33, 54.3153) centre (24.13, 54.3153) ccw
  arc A387 (23.33, 54.3153) -> (24.93, 54.3153) centre (24.13, 54.3153) ccw
  arc A388 (24.93, 56.8553) -> (23.33, 56.8553) centre (24.13, 56.8553) ccw
  arc A389 (23.33, 56.8553) -> (24.93, 56.8553) centre (24.13, 56.8553) ccw
  arc A390 (24.93, 56.8553) -> (23.33, 56.8553) centre (24.13, 56.8553) ccw
  arc A391 (23.33, 56.8553) -> (24.93, 56.8553) centre (24.13, 56.8553) ccw
  arc A392 (24.93, 56.8553) -> (23.33, 56.8553) centre (24.13, 56.8553) ccw
  arc A393 (23.33, 56.8553) -> (24.93, 56.8553) centre (24.13, 56.8553) ccw
  arc A394 (24.93, 59.3953) -> (23.33, 59.3953) centre (24.13, 59.3953) ccw
  arc A395 (23.33, 59.3953) -> (24.93, 59.3953) centre (24.13, 59.3953) ccw
  arc A396 (24.93, 59.3953) -> (23.33, 59.3953) centre (24.13, 59.3953) ccw
  arc A397 (23.33, 59.3953) -> (24.93, 59.3953) centre (24.13, 59.3953) ccw
  arc A398 (24.93, 59.3953) -> (23.33, 59.3953) centre (24.13, 59.3953) ccw
  arc A399 (23.33, 59.3953) -> (24.93, 59.3953) centre (24.13, 59.3953) ccw
  arc A400 (23.33, 61.9353) -> (24.93, 61.9353) centre (24.13, 61.9353) ccw
  arc A401 (24.93, 61.9353) -> (23.33, 61.9353) centre (24.13, 61.9353) ccw
  arc A402 (24.93, 61.9353) -> (23.33, 61.9353) centre (24.13, 61.9353) ccw
  arc A403 (23.33, 61.9353) -> (24.93, 61.9353) centre (24.13, 61.9353) ccw
  arc A404 (23.33, 61.9353) -> (24.93, 61.9353) centre (24.13, 61.9353) ccw
  arc A405 (24.93, 61.9353) -> (23.33, 61.9353) centre (24.13, 61.9353) ccw
  arc A406 (23.33, 64.4753) -> (24.93, 64.4753) centre (24.13, 64.4753) ccw
  arc A407 (24.93, 64.4753) -> (23.33, 64.4753) centre (24.13, 64.4753) ccw
  arc A408 (24.93, 64.4753) -> (23.33, 64.4753) centre (24.13, 64.4753) ccw
  arc A409 (23.33, 64.4753) -> (24.93, 64.4753) centre (24.13, 64.4753) ccw
  arc A410 (23.33, 64.4753) -> (24.93, 64.4753) centre (24.13, 64.4753) ccw
  arc A411 (24.93, 64.4753) -> (23.33, 64.4753) centre (24.13, 64.4753) ccw
  arc A412 (24.93, 67.0153) -> (23.33, 67.0153) centre (24.13, 67.0153) ccw
  arc A413 (23.33, 67.0153) -> (24.93, 67.0153) centre (24.13, 67.0153) ccw
  arc A414 (23.33, 67.0153) -> (24.93, 67.0153) centre (24.13, 67.0153) ccw
  arc A415 (24.93, 67.0153) -> (23.33, 67.0153) centre (24.13, 67.0153) ccw
  arc A416 (24.93, 67.0153) -> (23.33, 67.0153) centre (24.13, 67.0153) ccw
  arc A417 (23.33, 67.0153) -> (24.93, 67.0153) centre (24.13, 67.0153) ccw
  arc A418 (23.33, 69.5553) -> (24.93, 69.5553) centre (24.13, 69.5553) ccw
  arc A419 (24.93, 69.5553) -> (23.33, 69.5553) centre (24.13, 69.5553) ccw
  arc A420 (23.33, 69.5553) -> (24.93, 69.5553) centre (24.13, 69.5553) ccw
  arc A421 (24.93, 69.5553) -> (23.33, 69.5553) centre (24.13, 69.5553) ccw
  arc A422 (23.33, 69.5553) -> (24.93, 69.5553) centre (24.13, 69.5553) ccw
  arc A423 (24.93, 69.5553) -> (23.33, 69.5553) centre (24.13, 69.5553) ccw
  arc A424 (23.33, 72.0954) -> (24.93, 72.0954) centre (24.13, 72.0954) ccw
  arc A425 (24.93, 72.0954) -> (23.33, 72.0954) centre (24.13, 72.0954) ccw
  arc A426 (23.33, 72.0954) -> (24.93, 72.0954) centre (24.13, 72.0954) ccw
  arc A427 (24.93, 72.0954) -> (23.33, 72.0954) centre (24.13, 72.0954) ccw
  arc A428 (24.93, 72.0954) -> (23.33, 72.0954) centre (24.13, 72.0954) ccw
  arc A429 (23.33, 72.0954) -> (24.93, 72.0954) centre (24.13, 72.0954) ccw
  arc A430 (24.93, 74.6354) -> (23.33, 74.6354) centre (24.13, 74.6354) ccw
  arc A431 (23.33, 74.6354) -> (24.93, 74.6354) centre (24.13, 74.6354) ccw
  arc A432 (23.33, 74.6354) -> (24.93, 74.6354) centre (24.13, 74.6354) ccw
  arc A433 (24.93, 74.6354) -> (23.33, 74.6354) centre (24.13, 74.6354) ccw
  arc A434 (24.93, 74.6354) -> (23.33, 74.6354) centre (24.13, 74.6354) ccw
  arc A435 (23.33, 74.6354) -> (24.93, 74.6354) centre (24.13, 74.6354) ccw
  arc A436 (24.93, 77.1754) -> (23.33, 77.1754) centre (24.13, 77.1754) ccw
  arc A437 (23.33, 77.1754) -> (24.93, 77.1754) centre (24.13, 77.1754) ccw
  arc A438 (24.93, 77.1754) -> (23.33, 77.1754) centre (24.13, 77.1754) ccw
  arc A439 (23.33, 77.1754) -> (24.93, 77.1754) centre (24.13, 77.1754) ccw
  arc A440 (24.93, 77.1754) -> (23.33, 77.1754) centre (24.13, 77.1754) ccw
  arc A441 (23.33, 77.1754) -> (24.93, 77.1754) centre (24.13, 77.1754) ccw
  arc A442 (23.33, 79.7154) -> (24.93, 79.7154) centre (24.13, 79.7154) ccw
  arc A443 (24.93, 79.7154) -> (23.33, 79.7154) centre (24.13, 79.7154) ccw
  arc A444 (23.33, 79.7154) -> (24.93, 79.7154) centre (24.13, 79.7154) ccw
  arc A445 (24.93, 79.7154) -> (23.33, 79.7154) centre (24.13, 79.7154) ccw
  arc A446 (24.93, 79.7154) -> (23.33, 79.7154) centre (24.13, 79.7154) ccw
  arc A447 (23.33, 79.7154) -> (24.93, 79.7154) centre (24.13, 79.7154) ccw
  arc A448 (24.93, 82.2554) -> (23.33, 82.2554) centre (24.13, 82.2554) ccw
  arc A449 (23.33, 82.2554) -> (24.93, 82.2554) centre (24.13, 82.2554) ccw
  arc A450 (24.93, 82.2554) -> (23.33, 82.2554) centre (24.13, 82.2554) ccw
  arc A451 (23.33, 82.2554) -> (24.93, 82.2554) centre (24.13, 82.2554) ccw
  arc A452 (24.93, 82.2554) -> (23.33, 82.2554) centre (24.13, 82.2554) ccw
  arc A453 (23.33, 82.2554) -> (24.93, 82.2554) centre (24.13, 82.2554) ccw
  arc A454 (24.93, 84.7954) -> (23.33, 84.7954) centre (24.13, 84.7954) ccw
  arc A455 (23.33, 84.7954) -> (24.93, 84.7954) centre (24.13, 84.7954) ccw
  arc A456 (23.33, 84.7954) -> (24.93, 84.7954) centre (24.13, 84.7954) ccw
  arc A457 (24.93, 84.7954) -> (23.33, 84.7954) centre (24.13, 84.7954) ccw
  arc A458 (24.93, 84.7954) -> (23.33, 84.7954) centre (24.13, 84.7954) ccw
  arc A459 (23.33, 84.7954) -> (24.93, 84.7954) centre (24.13, 84.7954) ccw
  arc A460 (24.93, 87.3354) -> (23.33, 87.3354) centre (24.13, 87.3354) ccw
  arc A461 (23.33, 87.3354) -> (24.93, 87.3354) centre (24.13, 87.3354) ccw
  arc A462 (24.93, 87.3354) -> (23.33, 87.3354) centre (24.13, 87.3354) ccw
  arc A463 (23.33, 87.3354) -> (24.93, 87.3354) centre (24.13, 87.3354) ccw
  arc A464 (24.93, 87.3354) -> (23.33, 87.3354) centre (24.13, 87.3354) ccw
  arc A465 (23.33, 87.3354) -> (24.93, 87.3354) centre (24.13, 87.3354) ccw
  arc A466 (10.63, 39.0753) -> (12.23, 39.0753) centre (11.43, 39.0753) ccw
  arc A467 (12.23, 39.0753) -> (10.63, 39.0753) centre (11.43, 39.0753) ccw
  arc A468 (12.23, 39.0753) -> (10.63, 39.0753) centre (11.43, 39.0753) ccw
  arc A469 (10.63, 39.0753) -> (12.23, 39.0753) centre (11.43, 39.0753) ccw
  arc A470 (12.23, 39.0753) -> (10.63, 39.0753) centre (11.43, 39.0753) ccw
  arc A471 (10.63, 39.0753) -> (12.23, 39.0753) centre (11.43, 39.0753) ccw
  arc A472 (14.77, 39.0753) -> (13.17, 39.0753) centre (13.97, 39.0753) ccw
  arc A473 (13.17, 39.0753) -> (14.77, 39.0753) centre (13.97, 39.0753) ccw
  arc A474 (14.77, 39.0753) -> (13.17, 39.0753) centre (13.97, 39.0753) ccw
  arc A475 (13.17, 39.0753) -> (14.77, 39.0753) centre (13.97, 39.0753) ccw
  arc A476 (13.17, 39.0753) -> (14.77, 39.0753) centre (13.97, 39.0753) ccw
  arc A477 (14.77, 39.0753) -> (13.17, 39.0753) centre (13.97, 39.0753) ccw
  arc A478 (17.31, 39.0753) -> (15.71, 39.0753) centre (16.51, 39.0753) ccw
  arc A479 (15.71, 39.0753) -> (17.31, 39.0753) centre (16.51, 39.0753) ccw
  arc A480 (17.31, 39.0753) -> (15.71, 39.0753) centre (16.51, 39.0753) ccw
  arc A481 (15.71, 39.0753) -> (17.31, 39.0753) centre (16.51, 39.0753) ccw
  arc A482 (15.71, 39.0753) -> (17.31, 39.0753) centre (16.51, 39.0753) ccw
  arc A483 (17.31, 39.0753) -> (15.71, 39.0753) centre (16.51, 39.0753) ccw
  arc A484 (19.85, 39.0753) -> (18.25, 39.0753) centre (19.05, 39.0753) ccw
  arc A485 (18.25, 39.0753) -> (19.85, 39.0753) centre (19.05, 39.0753) ccw
  arc A486 (18.25, 39.0753) -> (19.85, 39.0753) centre (19.05, 39.0753) ccw
  arc A487 (19.85, 39.0753) -> (18.25, 39.0753) centre (19.05, 39.0753) ccw
  arc A488 (19.85, 39.0753) -> (18.25, 39.0753) centre (19.05, 39.0753) ccw
  arc A489 (18.25, 39.0753) -> (19.85, 39.0753) centre (19.05, 39.0753) ccw
  arc A490 (45.4661, 87.1512) -> (42.9261, 87.1512) centre (44.1961, 87.1512) ccw
  arc A491 (42.9261, 87.1512) -> (45.4661, 87.1512) centre (44.1961, 87.1512) ccw
  arc A492 (45.4661, 87.1512) -> (42.9261, 87.1512) centre (44.1961, 87.1512) ccw
  arc A493 (42.9261, 87.1512) -> (45.4661, 87.1512) centre (44.1961, 87.1512) ccw
  arc A494 (45.4661, 87.1512) -> (42.9261, 87.1512) centre (44.1961, 87.1512) ccw
  arc A495 (42.9261, 87.1512) -> (45.4661, 87.1512) centre (44.1961, 87.1512) ccw
  arc A496 (39.1161, 84.6112) -> (36.5761, 84.6112) centre (37.8461, 84.6112) ccw
  arc A497 (36.5761, 84.6112) -> (39.1161, 84.6112) centre (37.8461, 84.6112) ccw
  arc A498 (39.1161, 84.6112) -> (36.5761, 84.6112) centre (37.8461, 84.6112) ccw